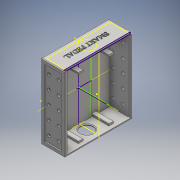
# Autodesk Inventor part: Part4
Saved by Autodesk Inventor 2016 (Build 200138000, 138)
## iProperties
Created: 2017-05-13
Part Number: Part4
Material: Generic
Document SubType Name: Modeling
Designer: ALIREZA
Density: 1 g/cm^3
Appearance: Default
Author: ALIREZA
Autodesk Inventor part; units mm, degrees
ref_plane "YZ Plane" through (0, 0, 0) normal (1, 0, 0) x (0, 1, 0)
ref_plane "XZ Plane" through (0, 0, 0) normal (0, 1, 0) x (-1, 0, 0)
ref_plane "XY Plane" through (0, 0, 0) normal (0, 0, 1) x (1, 0, 0)
sketch "Sketch1" plane through (0, 0, 0) normal (1, 0, 0) x (0, 1, 0)
  line L0 (50, 55) -> (-50, 55)
  line L1 (-50, 55) -> (-50, -55)
  line L2 (-50, -55) -> (50, -55)
  line L3 (50, -55) -> (50, 55)
  line L4 (50, 55) -> (-50, -55) construction
  line L5 (-50, 55) -> (50, -55) construction
  point P0 (0, 0)
  dimension "d0" = 100
  dimension "d1" = 110
  constraints: 12 end point, 2 midpoint, 2 parallel, 1 horizontal, 1 perpendicular
  measures "d0" distance of L2.end L1.end
  measures "d1" distance of L1.end L0.end
extrude "Extrusion1" add sketch "Sketch1" along normal blind 35
fillet "Fillet1" radius 1 12 edges at (17.5, 50, 55) (35, 50, 0) (35, 0, 55) (0, 0, 55) (0, 50, 0) (17.5, 50, -55) (35, 0, -55) (35, -50, 0) (17.5, -50, 55) (0, -50, 0) (0, 0, -55) (17.5, -50, -55)
sketch "Sketch2" plane through (35, 0, 0) normal (1, 0, 0) x (0, 0, -1)
  line L0 (52.5, -46.5) -> (-52.5, -46.5)
  line L1 (-52.5, -46.5) -> (-52.5, 46.5)
  line L2 (-52.5, 46.5) -> (52.5, 46.5)
  line L3 (52.5, 46.5) -> (52.5, -46.5)
  line L4 (52.5, -46.5) -> (-52.5, 46.5) construction
  line L5 (-52.5, -46.5) -> (52.5, 46.5) construction
  point P0 (0, 0)
  dimension "d5" = 105
  dimension "d6" = 93
  constraints: 12 end point, 2 midpoint, 2 parallel, 1 horizontal, 1 perpendicular
  measures "d5" distance of L1.end L2.end
  measures "d6" distance of L0.end L1.end
extrude "Extrusion2" cut sketch "Sketch2" against normal blind 30
sketch "Sketch3" plane through (34, 49, -55) normal (0, 0, -1) x (-1, 0, 0)
  line L0 (33, -98) -> (0, -98) projected
  line L1 (0, 0) -> (33, 0) projected
  circle A0 centre (16.5, -49) radius 9.5
  line L2 (16.5, -49) -> (16.5, -11.5096)
  line L3 (16.5, -49) -> (16.5, -84.2474)
  point P0 (34, -49)
  dimension "d55" = 19
  constraints: 4 end point, 2 vertical, 1 centre point
  measures "d55" diameter of A0
extrude "Extrusion3" cut sketch "Sketch3" against normal blind 30
sketch "Sketch4" plane through (0, 0, 0) normal (-1, 0, 0) x (0, 0, 1)
  point P0 (0, 0)
sketch "Sketch5" plane through (0, 0, 0) normal (-1, 0, 0) x (0, 0, 1)
  line L0 (19.6047, -32.8429) -> (51.5381, -32.8429) construction
  line L1 (51.5381, -32.8429) -> (51.5381, -46.3843) construction
  line L2 (51.5381, -46.3843) -> (19.6047, -46.3843) construction
  line L3 (19.6047, -46.3843) -> (19.6047, -32.8429) construction
  line L4 (20.2753, -38.9429) -> (20.2753, -32.8429)
  line L5 (20.2753, -32.8429) -> (21.532, -32.8429)
  line L6 (21.532, -32.8429) -> (21.532, -38.9429)
  line L7 (21.532, -38.9429) -> (20.2753, -38.9429)
  line L8 (22.8434, -38.9429) -> (22.8434, -32.8429)
  line L9 (22.8434, -32.8429) -> (24.7013, -32.8429)
  line L10 (24.7013, -32.8429) -> (25.9183, -37.4874)
  line L11 (25.9183, -37.4874) -> (27.1154, -32.8429)
  line L12 (27.1154, -32.8429) -> (28.9782, -32.8429)
  line L13 (28.9782, -32.8429) -> (28.9782, -38.9429)
  line L14 (28.9782, -38.9429) -> (27.8009, -38.9429)
  line L15 (27.8009, -38.9429) -> (27.8009, -34.0251)
  line L16 (27.8009, -34.0251) -> (26.564, -38.9429)
  line L17 (26.564, -38.9429) -> (25.2775, -38.9429)
  line L18 (25.2775, -38.9429) -> (24.0207, -34.0251)
  line L19 (24.0207, -34.0251) -> (24.0207, -38.9429)
  line L20 (24.0207, -38.9429) -> (22.8434, -38.9429)
  line L21 (31.5066, -38.9429) -> (31.5066, -33.9307)
  line L22 (31.5066, -33.9307) -> (29.6985, -33.9307)
  line L23 (29.6985, -33.9307) -> (29.6985, -32.8429)
  line L24 (29.6985, -32.8429) -> (34.5616, -32.8429)
  line L25 (34.5616, -32.8429) -> (34.5616, -33.9307)
  line L26 (34.5616, -33.9307) -> (32.7634, -33.9307)
  line L27 (32.7634, -33.9307) -> (32.7634, -38.9429)
  line L28 (32.7634, -38.9429) -> (31.5066, -38.9429)
  line L29 (35.2868, -38.9429) -> (35.2868, -32.8429)
  line L30 (35.2868, -32.8429) -> (39.7178, -32.8429)
  line L31 (39.7178, -32.8429) -> (39.7178, -33.9059)
  line L32 (39.7178, -33.9059) -> (36.5237, -33.9059)
  line L33 (36.5237, -33.9059) -> (36.5237, -35.2074)
  line L34 (36.5237, -35.2074) -> (39.4446, -35.2074)
  line L35 (39.4446, -35.2074) -> (39.4446, -36.2505)
  line L36 (39.4446, -36.2505) -> (36.5237, -36.2505)
  line L37 (36.5237, -36.2505) -> (36.5237, -37.8153)
  line L38 (36.5237, -37.8153) -> (39.8668, -37.8153)
  line L39 (39.8668, -37.8153) -> (39.8668, -38.9429)
  line L40 (39.8668, -38.9429) -> (35.2868, -38.9429)
  line L41 (40.8255, -38.9429) -> (40.8255, -32.8429)
  line L42 (40.8255, -32.8429) -> (42.0823, -32.8429)
  line L43 (42.0823, -32.8429) -> (42.0823, -35.3465)
  line L44 (42.0823, -35.3465) -> (44.4666, -32.8429)
  line L45 (44.4666, -32.8429) -> (46.0364, -32.8429)
  line L46 (46.0364, -32.8429) -> (43.5973, -35.3117)
  line L47 (43.5973, -35.3117) -> (46.2549, -38.9429)
  line L48 (46.2549, -38.9429) -> (44.72, -38.9429)
  line L49 (44.72, -38.9429) -> (42.733, -36.1512)
  line L50 (42.733, -36.1512) -> (42.0823, -36.797)
  line L51 (42.0823, -36.797) -> (42.0823, -38.9429)
  line L52 (42.0823, -38.9429) -> (40.8255, -38.9429)
  point P0 (0, 0)
  constraints: 2 other
sketch "Sketch6" plane through (0, 0, 0) normal (-1, 0, 0) x (0, 0, 1)
  point P0 (0, 0)
sketch "Sketch7" plane through (0, 0, 0) normal (-1, 0, 0) x (0, 0, 1)
  point P0 (0, 0)
sketch "Sketch8" plane through (0, 0, 0) normal (-1, 0, 0) x (0, 0, 1)
  point P0 (0, 0)
emboss "Emboss1" sketch "Sketch5" operation add depth 0.5 direction (1, 0, 0)
sketch "Sketch9" plane through (1, -49, 55) normal (0, 0, 1) x (1, 0, 0)
  line L0 (19.7914, 80.3195) -> (19.7914, -11.2085) construction
  line L1 (19.7914, -11.2085) -> (-27.1496, -11.2085) construction
  line L2 (-27.1496, -11.2085) -> (-27.1496, 80.3195) construction
  line L3 (-27.1496, 80.3195) -> (19.7914, 80.3195) construction
  line L4 (19.7914, 76.1011) -> (17.6889, 76.1011)
  line L5 (17.6889, 76.1011) -> (17.6889, 76.2685)
  spline S0 degree 2 poles (17.6889, 76.2685) (18.2915, 76.3488) (19.008, 76.764) (19.4365, 77.5407) (19.4365, 77.9492) knots 0 0 0 1 2 3 3 3
  spline S1 degree 2 poles (19.4365, 77.9492) (19.4365, 78.4179) (18.8607, 79.0272) (18.4991, 79.0272) knots 0 0 0 1 2 2 2
  spline S2 degree 2 poles (18.4991, 79.0272) (18.2178, 79.0272) (17.9902, 78.8397) knots 0 0 0 1 1 1
  spline S3 degree 2 poles (17.9902, 78.8397) (17.6487, 78.5585) (17.0862, 77.5072) knots 0 0 0 1 1 1
  spline S4 degree 2 poles (17.0862, 77.5072) (16.6309, 76.6568) (16.1421, 76.0341) (15.4725, 75.6993) (15.1109, 75.6993) knots 0 0 0 1 2 3 3 3
  spline S5 degree 2 poles (15.1109, 75.6993) (14.4213, 75.6993) (13.4169, 76.7707) (13.4169, 77.6144) knots 0 0 0 1 2 2 2
  spline S6 degree 2 poles (13.4169, 77.6144) (13.4169, 77.8822) (13.457, 78.1099) knots 0 0 0 1 1 1
  spline S7 degree 2 poles (13.457, 78.1099) (13.4838, 78.2505) (13.7651, 79.1276) (13.7651, 79.2482) knots 0 0 0 1 2 2 2
  spline S8 degree 2 poles (13.7651, 79.2482) (13.7651, 79.3553) (13.6244, 79.4892) (13.4169, 79.516) knots 0 0 0 1 2 2 2
  line L6 (13.4169, 79.516) -> (13.4169, 79.6834)
  line L7 (13.4169, 79.6834) -> (15.506, 79.6834)
  line L8 (15.506, 79.6834) -> (15.506, 79.516)
  spline S9 degree 2 poles (15.506, 79.516) (14.8498, 79.4022) (14.2003, 79.0071) (13.7651, 78.1969) (13.7651, 77.7081) knots 0 0 0 1 2 3 3 3
  spline S10 degree 2 poles (13.7651, 77.7081) (13.7651, 77.1523) (14.3677, 76.4961) (14.7627, 76.4961) knots 0 0 0 1 2 2 2
  spline S11 degree 2 poles (14.7627, 76.4961) (14.9904, 76.4961) (15.4524, 76.7439) (15.6466, 77.005) knots 0 0 0 1 2 2 2
  spline S12 degree 2 poles (15.6466, 77.005) (15.7805, 77.1791) (16.6577, 78.7393) (17.18, 79.4022) (17.8094, 79.7437) (18.1844, 79.7437) knots 0 0 0 1 2 3 4 4 4
  spline S13 degree 2 poles (18.1844, 79.7437) (18.8406, 79.7437) (19.7914, 78.7393) (19.7914, 77.9626) knots 0 0 0 1 2 2 2
  spline S14 degree 2 poles (19.7914, 77.9626) (19.7914, 77.4737) (19.557, 76.9314) knots 0 0 0 1 1 1
  spline S15 degree 2 poles (19.557, 76.9314) (19.4365, 76.6769) (19.4365, 76.5765) knots 0 0 0 1 1 1
  spline S16 degree 2 poles (19.4365, 76.5765) (19.4365, 76.456) (19.5771, 76.3154) (19.7914, 76.2685) knots 0 0 0 1 2 2 2
  line L9 (19.7914, 76.2685) -> (19.7914, 76.1011)
  line L10 (13.5575, 71.4273) -> (18.6866, 73.7843)
  line L11 (18.6866, 73.7843) -> (14.6154, 73.7843)
  spline S17 degree 2 poles (14.6154, 73.7843) (14.053, 73.7843) (13.9124, 73.6638) knots 0 0 0 1 1 1
  spline S18 degree 2 poles (13.9124, 73.6638) (13.7249, 73.4964) (13.7249, 73.1415) knots 0 0 0 1 1 1
  line L12 (13.7249, 73.1415) -> (13.7249, 72.9205)
  line L13 (13.7249, 72.9205) -> (13.5575, 72.9205)
  line L14 (13.5575, 72.9205) -> (13.5575, 75.0431)
  line L15 (13.5575, 75.0431) -> (13.7249, 75.0431)
  line L16 (13.7249, 75.0431) -> (13.7249, 74.8289)
  spline S19 degree 2 poles (13.7249, 74.8289) (13.7249, 74.4405) (13.9592, 74.2798) knots 0 0 0 1 1 1
  spline S20 degree 2 poles (13.9592, 74.2798) (14.1065, 74.1793) (14.6154, 74.1793) knots 0 0 0 1 1 1
  line L17 (14.6154, 74.1793) -> (18.5995, 74.1793)
  spline S21 degree 2 poles (18.5995, 74.1793) (19.0013, 74.1793) (19.1754, 74.2731) knots 0 0 0 1 1 1
  spline S22 degree 2 poles (19.1754, 74.2731) (19.3093, 74.3334) (19.4834, 74.6682) (19.4834, 75.0431) knots 0 0 0 1 2 2 2
  line L18 (19.4834, 75.0431) -> (19.6575, 75.0431)
  line L19 (19.6575, 75.0431) -> (19.6575, 73.3156)
  line L20 (19.6575, 73.3156) -> (14.8833, 71.1059)
  line L21 (14.8833, 71.1059) -> (19.6575, 68.9297)
  line L22 (19.6575, 68.9297) -> (19.6575, 67.2089)
  line L23 (19.6575, 67.2089) -> (19.4834, 67.2089)
  line L24 (19.4834, 67.2089) -> (19.4834, 67.4164)
  spline S23 degree 2 poles (19.4834, 67.4164) (19.4834, 67.8115) (19.2557, 67.9655) knots 0 0 0 1 1 1
  spline S24 degree 2 poles (19.2557, 67.9655) (19.1084, 68.066) (18.5995, 68.066) knots 0 0 0 1 1 1
  line L25 (18.5995, 68.066) -> (14.6154, 68.066)
  spline S25 degree 2 poles (14.6154, 68.066) (14.053, 68.066) (13.9124, 67.9454) knots 0 0 0 1 1 1
  spline S26 degree 2 poles (13.9124, 67.9454) (13.7249, 67.778) (13.7249, 67.4164) knots 0 0 0 1 1 1
  line L26 (13.7249, 67.4164) -> (13.7249, 67.2089)
  line L27 (13.7249, 67.2089) -> (13.5575, 67.2089)
  line L28 (13.5575, 67.2089) -> (13.5575, 69.8002)
  line L29 (13.5575, 69.8002) -> (13.7249, 69.8002)
  line L30 (13.7249, 69.8002) -> (13.7249, 69.5792)
  spline S27 degree 2 poles (13.7249, 69.5792) (13.7249, 69.1842) (13.9592, 69.0302) knots 0 0 0 1 1 1
  spline S28 degree 2 poles (13.9592, 69.0302) (14.1065, 68.9297) (14.6154, 68.9297) knots 0 0 0 1 1 1
  line L31 (14.6154, 68.9297) -> (18.6866, 68.9297)
  line L32 (18.6866, 68.9297) -> (13.5575, 71.2867)
  line L33 (13.5575, 71.2867) -> (13.5575, 71.4273)
  line L34 (15.593, 62.8029) -> (15.593, 65.1599)
  line L35 (15.593, 65.1599) -> (14.6355, 65.5751)
  spline S29 degree 2 poles (14.6355, 65.5751) (14.2806, 65.7291) (14.1065, 65.7291) knots 0 0 0 1 1 1
  spline S30 degree 2 poles (14.1065, 65.7291) (13.9659, 65.7291) (13.7517, 65.4612) (13.7249, 65.026) knots 0 0 0 1 2 2 2
  line L36 (13.7249, 65.026) -> (13.5575, 65.026)
  line L37 (13.5575, 65.026) -> (13.5575, 66.9477)
  line L38 (13.5575, 66.9477) -> (13.7249, 66.9477)
  spline S31 degree 2 poles (13.7249, 66.9477) (13.7918, 66.5594) (13.899, 66.4455) knots 0 0 0 1 1 1
  spline S32 degree 2 poles (13.899, 66.4455) (14.1132, 66.2179) (14.7761, 65.9433) knots 0 0 0 1 1 1
  line L39 (14.7761, 65.9433) -> (19.7914, 63.8006)
  line L40 (19.7914, 63.8006) -> (19.7914, 63.6399)
  line L41 (19.7914, 63.6399) -> (14.7159, 61.5173)
  spline S33 degree 2 poles (14.7159, 61.5173) (14.1065, 61.2629) (13.7517, 60.841) (13.7249, 60.4728) knots 0 0 0 1 2 2 2
  line L42 (13.7249, 60.4728) -> (13.5575, 60.4728)
  line L43 (13.5575, 60.4728) -> (13.5575, 62.8766)
  line L44 (13.5575, 62.8766) -> (13.7249, 62.8766)
  spline S34 degree 2 poles (13.7249, 62.8766) (13.745, 62.5083) (13.9458, 62.2539) (14.0998, 62.2539) knots 0 0 0 1 2 2 2
  spline S35 degree 2 poles (14.0998, 62.2539) (14.294, 62.2539) (14.7159, 62.4347) knots 0 0 0 1 1 1
  line L45 (14.7159, 62.4347) -> (15.593, 62.8029)
  line L46 (15.9345, 62.9235) -> (18.3919, 63.9613)
  line L47 (18.3919, 63.9613) -> (15.9345, 65.026)
  line L48 (15.9345, 65.026) -> (15.9345, 62.9235)
  line L49 (13.5575, 54.1451) -> (13.5575, 55.7722)
  line L50 (13.5575, 55.7722) -> (16.4099, 57.8346)
  spline S36 degree 2 poles (16.4099, 57.8346) (16.3966, 58.0689) (16.3966, 58.2028) knots 0 0 0 1 1 1
  spline S37 degree 2 poles (16.3966, 58.2028) (16.3966, 58.2698) (16.4032, 58.4037) (16.4099, 58.4707) knots 0 0 0 1 2 2 2
  line L51 (16.4099, 58.4707) -> (14.6355, 58.4707)
  spline S38 degree 2 poles (14.6355, 58.4707) (14.0597, 58.4707) (13.9258, 58.3435) knots 0 0 0 1 1 1
  spline S39 degree 2 poles (13.9258, 58.3435) (13.7249, 58.1761) (13.7249, 57.8346) knots 0 0 0 1 1 1
  line L52 (13.7249, 57.8346) -> (13.7249, 57.5935)
  line L53 (13.7249, 57.5935) -> (13.5575, 57.5935)
  line L54 (13.5575, 57.5935) -> (13.5575, 60.2116)
  line L55 (13.5575, 60.2116) -> (13.7249, 60.2116)
  line L56 (13.7249, 60.2116) -> (13.7249, 59.9773)
  spline S40 degree 2 poles (13.7249, 59.9773) (13.7249, 59.5956) (13.9726, 59.4282) knots 0 0 0 1 1 1
  spline S41 degree 2 poles (13.9726, 59.4282) (14.1132, 59.3345) (14.6355, 59.3345) knots 0 0 0 1 1 1
  line L57 (14.6355, 59.3345) -> (18.5727, 59.3345)
  spline S42 degree 2 poles (18.5727, 59.3345) (19.1486, 59.3345) (19.2892, 59.4617) knots 0 0 0 1 1 1
  spline S43 degree 2 poles (19.2892, 59.4617) (19.4834, 59.6358) (19.4834, 59.9773) knots 0 0 0 1 1 1
  line L58 (19.4834, 59.9773) -> (19.4834, 60.2116)
  line L59 (19.4834, 60.2116) -> (19.6575, 60.2116)
  line L60 (19.6575, 60.2116) -> (19.6575, 57.9886)
  spline S44 degree 2 poles (19.6575, 57.9886) (19.6575, 57.0177) (19.3696, 56.1003) (18.6062, 55.4508) (18.0839, 55.4508) knots 0 0 0 1 2 3 3 3
  spline S45 degree 2 poles (18.0839, 55.4508) (17.5215, 55.4508) (16.6912, 56.1874) (16.5238, 56.9574) knots 0 0 0 1 2 2 2
  line L61 (16.5238, 56.9574) -> (14.7761, 55.6986)
  spline S46 degree 2 poles (14.7761, 55.6986) (14.1735, 55.27) (13.7784, 54.6473) (13.7249, 54.1451) knots 0 0 0 1 2 2 2
  line L62 (13.7249, 54.1451) -> (13.5575, 54.1451)
  spline S47 degree 2 poles (16.6845, 58.4707) (16.6845, 58.3836) (16.6845, 58.2631) (16.6845, 58.2229) knots 0 0 0 1 2 2 2
  spline S48 degree 2 poles (16.6845, 58.2229) (16.6845, 57.3525) (17.4411, 56.4619) (18.0237, 56.4619) knots 0 0 0 1 2 2 2
  spline S49 degree 2 poles (18.0237, 56.4619) (18.5995, 56.4619) (19.3093, 57.1784) (19.3093, 57.7676) knots 0 0 0 1 2 2 2
  spline S50 degree 2 poles (19.3093, 57.7676) (19.3093, 58.0287) (19.2222, 58.4707) knots 0 0 0 1 1 1
  line L63 (19.2222, 58.4707) -> (16.6845, 58.4707)
  line L64 (19.6575, 48.9022) -> (18.2178, 48.8285)
  line L65 (18.2178, 48.8285) -> (18.2178, 49.0026)
  spline S51 degree 2 poles (18.2178, 49.0026) (18.5995, 49.0495) (18.7602, 49.1365) knots 0 0 0 1 1 1
  spline S52 degree 2 poles (18.7602, 49.1365) (19.0214, 49.2772) (19.2691, 49.7459) (19.2691, 50.1208) knots 0 0 0 1 2 2 2
  line L66 (19.2691, 50.1208) -> (19.2691, 50.9712)
  line L67 (19.2691, 50.9712) -> (14.6154, 50.9712)
  spline S53 degree 2 poles (14.6154, 50.9712) (14.053, 50.9712) (13.9124, 50.8507) knots 0 0 0 1 1 1
  spline S54 degree 2 poles (13.9124, 50.8507) (13.7249, 50.6833) (13.7249, 50.3284) knots 0 0 0 1 1 1
  line L68 (13.7249, 50.3284) -> (13.7249, 50.1208)
  line L69 (13.7249, 50.1208) -> (13.5575, 50.1208)
  line L70 (13.5575, 50.1208) -> (13.5575, 52.7055)
  line L71 (13.5575, 52.7055) -> (13.7249, 52.7055)
  line L72 (13.7249, 52.7055) -> (13.7249, 52.4845)
  spline S55 degree 2 poles (13.7249, 52.4845) (13.7249, 52.1028) (13.9592, 51.9354) knots 0 0 0 1 1 1
  spline S56 degree 2 poles (13.9592, 51.9354) (14.1065, 51.8417) (14.6154, 51.8417) knots 0 0 0 1 1 1
  line L73 (14.6154, 51.8417) -> (19.2691, 51.8417)
  line L74 (19.2691, 51.8417) -> (19.2691, 52.5716)
  spline S57 degree 2 poles (19.2691, 52.5716) (19.2691, 53.0001) (19.2088, 53.1809) knots 0 0 0 1 1 1
  spline S58 degree 2 poles (19.2088, 53.1809) (19.1218, 53.4152) (18.6397, 53.7433) (18.2178, 53.7768) knots 0 0 0 1 2 2 2
  line L75 (18.2178, 53.7768) -> (18.2178, 53.9442)
  line L76 (18.2178, 53.9442) -> (19.6575, 53.8773)
  line L77 (19.6575, 53.8773) -> (19.6575, 48.9022)
  line L78 (16.4099, 44.4226) -> (14.6355, 44.4226)
  spline S59 degree 2 poles (14.6355, 44.4226) (14.0597, 44.4226) (13.9258, 44.2954) knots 0 0 0 1 1 1
  spline S60 degree 2 poles (13.9258, 44.2954) (13.7249, 44.128) (13.7249, 43.7798) knots 0 0 0 1 1 1
  line L79 (13.7249, 43.7798) -> (13.7249, 43.5454)
  line L80 (13.7249, 43.5454) -> (13.5575, 43.5454)
  line L81 (13.5575, 43.5454) -> (13.5575, 46.1568)
  line L82 (13.5575, 46.1568) -> (13.7249, 46.1568)
  line L83 (13.7249, 46.1568) -> (13.7249, 45.9292)
  spline S61 degree 2 poles (13.7249, 45.9292) (13.7249, 45.5475) (13.9726, 45.3734) knots 0 0 0 1 1 1
  spline S62 degree 2 poles (13.9726, 45.3734) (14.1132, 45.2864) (14.6355, 45.2864) knots 0 0 0 1 1 1
  line L84 (14.6355, 45.2864) -> (18.5727, 45.2864)
  spline S63 degree 2 poles (18.5727, 45.2864) (19.1486, 45.2864) (19.2892, 45.4069) knots 0 0 0 1 1 1
  spline S64 degree 2 poles (19.2892, 45.4069) (19.4834, 45.5877) (19.4834, 45.9292) knots 0 0 0 1 1 1
  line L85 (19.4834, 45.9292) -> (19.4834, 46.1568)
  line L86 (19.4834, 46.1568) -> (19.6575, 46.1568)
  line L87 (19.6575, 46.1568) -> (19.6575, 43.9271)
  spline S65 degree 2 poles (19.6575, 43.9271) (19.6575, 43.1035) (19.3093, 42.1661) (18.5192, 41.5166) (17.9634, 41.5166) knots 0 0 0 1 2 3 3 3
  spline S66 degree 2 poles (17.9634, 41.5166) (17.2202, 41.5166) (16.2894, 42.5009) (16.2894, 43.3981) knots 0 0 0 1 2 2 2
  spline S67 degree 2 poles (16.2894, 43.3981) (16.2894, 43.6191) (16.3497, 44.1347) (16.4099, 44.4226) knots 0 0 0 1 2 2 2
  spline S68 degree 2 poles (16.6711, 44.4226) (16.6242, 44.1882) (16.5773, 43.8133) (16.5773, 43.686) knots 0 0 0 1 2 2 2
  spline S69 degree 2 poles (16.5773, 43.686) (16.5773, 43.2173) (17.3005, 42.541) (17.8764, 42.541) knots 0 0 0 1 2 2 2
  spline S70 degree 2 poles (17.8764, 42.541) (18.2714, 42.541) (18.9544, 42.8624) (19.2892, 43.4584) (19.2892, 43.84) knots 0 0 0 1 2 3 3 3
  spline S71 degree 2 poles (19.2892, 43.84) (19.2892, 44.061) (19.2022, 44.4226) knots 0 0 0 1 1 1
  line L88 (19.2022, 44.4226) -> (16.6711, 44.4226)
  line L89 (19.316, 39.2667) -> (16.9054, 39.2667)
  line L90 (16.9054, 39.2667) -> (16.9054, 37.9275)
  spline S72 degree 2 poles (16.9054, 37.9275) (16.9054, 37.4053) (17.0661, 37.2312) knots 0 0 0 1 1 1
  spline S73 degree 2 poles (17.0661, 37.2312) (17.2737, 36.9968) (17.796, 36.97) knots 0 0 0 1 1 1
  line L91 (17.796, 36.97) -> (17.796, 36.8026)
  line L92 (17.796, 36.8026) -> (15.6801, 36.8026)
  line L93 (15.6801, 36.8026) -> (15.6801, 36.97)
  spline S74 degree 2 poles (15.6801, 36.97) (16.1153, 37.0303) (16.2492, 37.0972) knots 0 0 0 1 1 1
  spline S75 degree 2 poles (16.2492, 37.0972) (16.4032, 37.1776) (16.584, 37.5392) (16.584, 37.9275) knots 0 0 0 1 2 2 2
  line L94 (16.584, 37.9275) -> (16.584, 39.2667)
  line L95 (16.584, 39.2667) -> (14.5753, 39.2667)
  spline S76 degree 2 poles (14.5753, 39.2667) (14.1668, 39.2667) (13.9927, 39.1931) (13.8856, 39.0123) (13.8856, 38.7645) knots 0 0 0 1 2 3 3 3
  line L96 (13.8856, 38.7645) -> (13.8856, 37.7267)
  spline S77 degree 2 poles (13.8856, 37.7267) (13.8856, 37.2111) (14.0329, 36.7491) (14.2405, 36.5281) knots 0 0 0 1 2 2 2
  spline S78 degree 2 poles (14.2405, 36.5281) (14.5217, 36.2469) (15.0841, 35.9589) knots 0 0 0 1 1 1
  line L97 (15.0841, 35.9589) -> (15.0841, 35.7781)
  line L98 (15.0841, 35.7781) -> (13.5575, 36.3071)
  line L99 (13.5575, 36.3071) -> (13.5575, 40.9943)
  line L100 (13.5575, 40.9943) -> (13.7249, 40.9943)
  line L101 (13.7249, 40.9943) -> (13.7249, 40.78)
  spline S79 degree 2 poles (13.7249, 40.78) (13.7249, 40.5657) (13.8253, 40.3782) knots 0 0 0 1 1 1
  spline S80 degree 2 poles (13.8253, 40.3782) (13.899, 40.2309) (14.1869, 40.1238) (14.6288, 40.1238) knots 0 0 0 1 2 2 2
  line L102 (14.6288, 40.1238) -> (18.5928, 40.1238)
  spline S81 degree 2 poles (18.5928, 40.1238) (19.1754, 40.1238) (19.3093, 40.2443) knots 0 0 0 1 1 1
  spline S82 degree 2 poles (19.3093, 40.2443) (19.4834, 40.405) (19.4834, 40.78) knots 0 0 0 1 1 1
  line L103 (19.4834, 40.78) -> (19.4834, 40.9943)
  line L104 (19.4834, 40.9943) -> (19.6575, 40.9943)
  line L105 (19.6575, 40.9943) -> (19.6575, 36.3071)
  line L106 (19.6575, 36.3071) -> (18.3183, 36.2335)
  line L107 (18.3183, 36.2335) -> (18.3183, 36.4076)
  spline S83 degree 2 poles (18.3183, 36.4076) (18.7937, 36.5013) (19.1553, 36.7357) (19.2557, 36.9633) knots 0 0 0 1 2 2 2
  spline S84 degree 2 poles (19.2557, 36.9633) (19.316, 37.1441) (19.316, 37.5927) knots 0 0 0 1 1 1
  line L108 (19.316, 37.5927) -> (19.316, 39.2667)
  line L109 (13.5575, 35.4166) -> (13.7249, 35.4166)
  line L110 (13.7249, 35.4166) -> (13.7249, 35.1822)
  spline S85 degree 2 poles (13.7249, 35.1822) (13.7249, 34.8005) (13.9726, 34.6331) knots 0 0 0 1 1 1
  spline S86 degree 2 poles (13.9726, 34.6331) (14.1199, 34.5394) (14.6355, 34.5394) knots 0 0 0 1 1 1
  line L111 (14.6355, 34.5394) -> (18.5727, 34.5394)
  spline S87 degree 2 poles (18.5727, 34.5394) (19.1419, 34.5394) (19.2892, 34.6666) knots 0 0 0 1 1 1
  spline S88 degree 2 poles (19.2892, 34.6666) (19.4834, 34.8407) (19.4834, 35.1822) knots 0 0 0 1 1 1
  line L112 (19.4834, 35.1822) -> (19.4834, 35.4166)
  line L113 (19.4834, 35.4166) -> (19.6575, 35.4166)
  line L114 (19.6575, 35.4166) -> (19.6575, 32.9324)
  spline S89 degree 2 poles (19.6575, 32.9324) (19.6575, 31.5664) (19.0348, 30.1402) (17.5884, 29.2764) (16.6376, 29.2764) knots 0 0 0 1 2 3 3 3
  spline S90 degree 2 poles (16.6376, 29.2764) (15.3654, 29.2764) (14.5083, 30.0464) knots 0 0 0 1 1 1
  spline S91 degree 2 poles (14.5083, 30.0464) (13.5575, 30.9169) (13.5575, 32.6913) knots 0 0 0 1 1 1
  line L115 (13.5575, 32.6913) -> (13.5575, 35.4166)
  spline S92 degree 2 poles (13.9994, 33.6689) (13.8722, 33.0998) (13.8722, 32.7181) knots 0 0 0 1 1 1
  spline S93 degree 2 poles (13.8722, 32.7181) (13.8722, 31.6735) (15.3386, 30.3009) (16.5907, 30.3009) knots 0 0 0 1 2 2 2
  spline S94 degree 2 poles (16.5907, 30.3009) (17.8563, 30.3009) (19.3093, 31.6735) (19.3093, 32.7516) knots 0 0 0 1 2 2 2
  spline S95 degree 2 poles (19.3093, 32.7516) (19.3093, 33.1533) (19.1754, 33.6689) knots 0 0 0 1 1 1
  line L116 (19.1754, 33.6689) -> (13.9994, 33.6689)
  line L117 (15.593, 24.7098) -> (15.593, 27.0667)
  line L118 (15.593, 27.0667) -> (14.6355, 27.4819)
  spline S96 degree 2 poles (14.6355, 27.4819) (14.2806, 27.6359) (14.1065, 27.6359) knots 0 0 0 1 1 1
  spline S97 degree 2 poles (14.1065, 27.6359) (13.9659, 27.6359) (13.7517, 27.368) (13.7249, 26.9328) knots 0 0 0 1 2 2 2
  line L119 (13.7249, 26.9328) -> (13.5575, 26.9328)
  line L120 (13.5575, 26.9328) -> (13.5575, 28.8545)
  line L121 (13.5575, 28.8545) -> (13.7249, 28.8545)
  spline S98 degree 2 poles (13.7249, 28.8545) (13.7918, 28.4662) (13.899, 28.3523) knots 0 0 0 1 1 1
  spline S99 degree 2 poles (13.899, 28.3523) (14.1132, 28.1247) (14.7761, 27.8501) knots 0 0 0 1 1 1
  line L122 (14.7761, 27.8501) -> (19.7914, 25.7074)
  line L123 (19.7914, 25.7074) -> (19.7914, 25.5467)
  line L124 (19.7914, 25.5467) -> (14.7159, 23.4241)
  spline S100 degree 2 poles (14.7159, 23.4241) (14.1065, 23.1697) (13.7517, 22.7478) (13.7249, 22.3796) knots 0 0 0 1 2 2 2
  line L125 (13.7249, 22.3796) -> (13.5575, 22.3796)
  line L126 (13.5575, 22.3796) -> (13.5575, 24.7834)
  line L127 (13.5575, 24.7834) -> (13.7249, 24.7834)
  spline S101 degree 2 poles (13.7249, 24.7834) (13.745, 24.4151) (13.9458, 24.1607) (14.0998, 24.1607) knots 0 0 0 1 2 2 2
  spline S102 degree 2 poles (14.0998, 24.1607) (14.294, 24.1607) (14.7159, 24.3415) knots 0 0 0 1 1 1
  line L128 (14.7159, 24.3415) -> (15.593, 24.7098)
  line L129 (15.9345, 24.8303) -> (18.3919, 25.8681)
  line L130 (18.3919, 25.8681) -> (15.9345, 26.9328)
  line L131 (15.9345, 26.9328) -> (15.9345, 24.8303)
  line L132 (15.2382, 16.996) -> (15.2114, 16.8487)
  line L133 (15.2114, 16.8487) -> (13.5575, 17.371)
  line L134 (13.5575, 17.371) -> (13.5575, 22.0849)
  line L135 (13.5575, 22.0849) -> (13.7249, 22.0849)
  line L136 (13.7249, 22.0849) -> (13.7249, 21.8573)
  spline S103 degree 2 poles (13.7249, 21.8573) (13.7249, 21.4689) (13.9726, 21.3082) knots 0 0 0 1 1 1
  spline S104 degree 2 poles (13.9726, 21.3082) (14.1199, 21.2078) (14.6422, 21.2078) knots 0 0 0 1 1 1
  line L137 (14.6422, 21.2078) -> (18.5727, 21.2078)
  spline S105 degree 2 poles (18.5727, 21.2078) (19.1419, 21.2078) (19.2892, 21.335) knots 0 0 0 1 1 1
  spline S106 degree 2 poles (19.2892, 21.335) (19.4834, 21.5091) (19.4834, 21.8573) knots 0 0 0 1 1 1
  line L138 (19.4834, 21.8573) -> (19.4834, 22.0849)
  line L139 (19.4834, 22.0849) -> (19.6575, 22.0849)
  line L140 (19.6575, 22.0849) -> (19.6575, 19.3262)
  line L141 (19.6575, 19.3262) -> (19.4834, 19.3262)
  spline S107 degree 2 poles (19.4834, 19.3262) (19.4901, 19.815) (19.3026, 20.2034) (19.0147, 20.3507) (18.4723, 20.3507) knots 0 0 0 1 2 3 3 3
  line L142 (18.4723, 20.3507) -> (14.6422, 20.3507)
  spline S108 degree 2 poles (14.6422, 20.3507) (14.2672, 20.3507) (14.1266, 20.277) knots 0 0 0 1 1 1
  spline S109 degree 2 poles (14.1266, 20.277) (14.0329, 20.2235) (13.9458, 19.9958) (13.9458, 19.4066) knots 0 0 0 1 2 2 2
  line L143 (13.9458, 19.4066) -> (13.9458, 18.9646)
  spline S110 degree 2 poles (13.9458, 18.9646) (13.9458, 18.2683) (14.1467, 17.6991) (14.6757, 17.2304) (15.2382, 16.996) knots 0 0 0 1 2 3 3 3
  point P0 (-1, 49)
  constraints: 2 other
emboss "Emboss2" sketch "Sketch9" operation add depth 0.5 direction (0, 0, -1)
sketch "Sketch10" plane through (1, -50, -54) normal (0, -1, 0) x (1, 0, 0)
  circle A0 centre (23.8045, 92.5062) radius 2.2175
  line L0 (23.8045, 92.5062) -> (31.7537, 92.5062)
  line L1 (31.7537, 92.5062) -> (18.4963, 92.5062)
  line L2 (18.4963, 92.5062) -> (23.8045, 92.5062)
  line L3 (24.7351, 104.1704) -> (24.7351, 90.393)
  line L4 (0, 108) -> (33, 108) projected
  circle A1 centre (23.8045, 72.9922) radius 2.2175
  circle A2 centre (23.8045, 53.4782) radius 2.2175
  circle A3 centre (23.8045, 33.9642) radius 2.2175
  circle A4 centre (23.8045, 14.4502) radius 2.2175
  circle A5 centre (9.1955, 92.5062) radius 2.2175
  circle A6 centre (9.1955, 72.9922) radius 2.2175
  circle A7 centre (9.1955, 53.4782) radius 2.2175
  circle A8 centre (9.1955, 33.9642) radius 2.2175
  circle A9 centre (9.1955, 14.4502) radius 2.2175
  line L5 (0, 0) -> (0, 108) projected
  line L6 (33, 108) -> (33, 0) projected
  line L7 (29, 103.2061) -> (4, 4.7939) construction
  line L8 (5.4125, 97.6458) -> (27.5875, 10.3542) construction
  point P0 (-1, 54)
  point P1 (16.5, 54)
  dimension "d15" = 4.435
  dimension "d26" = 19.514
  dimension "d33" = 19.514
  constraints: 12 end point, 10 centre point, 2 midpoint, 1 collinear, 1 horizontal, 1 perpendicular, 1 point on line, 1 vertical, 8 other
  measures "d15" diameter of A0
  measures "d26" distance of L0.start A1.centre
  measures "d33" distance of A6.centre A5.centre
extrude "Extrusion4" cut sketch "Sketch10" against normal blind 200
sketch "Sketch11" plane through (1, -50, -54) normal (0, -1, 0) x (1, 0, 0)
  point P0 (-1, 54)
sketch "Sketch12" plane through (1, -50, -54) normal (0, -1, 0) x (1, 0, 0)
  point P0 (-1, 54)
sketch "Sketch13" plane through (1, -50, -54) normal (0, -1, 0) x (1, 0, 0)
  point P0 (-1, 54)
sketch "Sketch14" plane through (35, -46.5, 52.5) normal (0, 1, 0) x (1, 0, 0)
  point P0 (-35, 52.5)
sketch "Sketch15" plane through (1, 50, 54) normal (0, 1, 0) x (1, 0, 0)
  line L0 (33, 108) -> (0, 108) projected
  line L1 (0, 108) -> (0, 0) projected
  line L2 (33, 108) -> (0, 108)
  line L3 (0, 108) -> (0, 0)
  line L4 (0, 0) -> (33, 0)
  line L5 (33, 0) -> (33, 108)
  line L6 (4, 106.5) -> (4, 1.5) projected
  line L7 (29, 103.6928) -> (4, 103.6928)
  line L8 (4, 103.6928) -> (4, 4.3072)
  line L9 (4, 4.3072) -> (29, 4.3072)
  line L10 (29, 4.3072) -> (29, 103.6928)
  line L11 (29, 103.6928) -> (4, 4.3072) construction
  line L12 (4, 103.6928) -> (29, 4.3072) construction
  point P0 (-1, 54)
  point P1 (16.5, 54)
  constraints: 20 end point, 4 parallel, 2 horizontal, 2 midpoint, 2 perpendicular, 1 point on line
extrude "Extrusion5" cut sketch "Sketch15" against normal blind 1.5 contours L7 L10 L9 L6
sketch "Sketch16" plane through (1, 48.5, 54) normal (0, 1, 0) x (1, 0, 0)
  point P0 (-1, 54)
sketch "Sketch17" plane through (5, 0, 0) normal (1, 0, 0) x (0, 0, -1)
  point P0 (0, 0)
sketch "Sketch18" plane through (5, 0, 0) normal (1, 0, 0) x (0, 0, -1)
  line L0 (52.5, -9.5) -> (52.5, 9.5) projected
  line L1 (52.5, 0) -> (-52.5, 0)
  line L2 (-52.5, -46.5) -> (-52.5, 46.5) projected
  point P0 (0, 0)
  constraints: 2 end point, 2 midpoint
ref_plane "Work Plane1" through (5, 0, -52.5) normal (0, 1, 0) x (0, 0, 1)
mirror "Mirror1" about plane through (5, 0, -52.5) normal (0, 1, 0) of "Extrusion5"
ref_plane "Work Plane2" through (2.5, 0, 0) normal (1, 0, 0) x (0, 0, -1)
ref_plane "Work Plane3" through (17.5, -49, 55) normal (1, 0, 0) x (0, 0, -1)
pattern_of_nothing "Mirror2"
sketch "Sketch19" plane through (1, -49, 55) normal (0, 0, 1) x (1, 0, 0)
  point P0 (-1, 49)
sketch "Sketch20" plane through (1, -49, 55) normal (0, 0, 1) x (1, 0, 0)
  point P0 (-1, 49)
sketch "Sketch21" plane through (32.5, 0, 0) normal (-1, 0, 0) x (0, 0, -1)
  point P0 (0, 0)
sketch "Sketch22" plane through (1, -49, 55) normal (0, 0, 1) x (1, 0, 0)
  point P0 (-1, 49)
sketch "Sketch23" plane through (1, -49, 55) normal (0, 0, 1) x (1, 0, 0)
  line L0 (33, 98) -> (0, 98) projected
  line L1 (0, 0) -> (33, 0) projected
  line L2 (33, 98) -> (31.1, 98)
  line L3 (31.1, 98) -> (31.1, 0)
  line L4 (31.1, 0) -> (33, 0)
  line L5 (33, 0) -> (33, 98)
  point P0 (-1, 49)
  dimension "d37" = 1.9
  constraints: 8 end point, 2 parallel, 1 horizontal, 1 perpendicular, 1 point on line
  measures "d37" distance of L4.end L3.end
extrude "Extrusion6" cut sketch "Sketch23" against normal up to surface (107.5 mm away)
sketch "Sketch24" plane through (35, 46.5, -52.5) normal (0, -1, 0) x (1, 0, 0)
  point P0 (-35, 52.5)
sketch "Sketch25" plane through (1, -49, 55) normal (0, 0, 1) x (1, 0, 0)
  point P0 (-1, 49)
sketch "Sketch26" plane through (1, -49, 55) normal (0, 0, 1) x (1, 0, 0)
  line L0 (34, 0) -> (34, 98) projected
  line L1 (31.1, 95.5) -> (31.1, 2.5) projected
  line L2 (34, 95.5519) -> (31.1, 95.5519)
  line L3 (31.1, 95.5519) -> (31.1, 2.5)
  line L4 (31.1, 2.5) -> (34, 2.5)
  line L5 (34, 2.5) -> (34, 95.5519)
  point P0 (-1, 49)
  constraints: 8 end point, 2 parallel, 1 horizontal, 1 perpendicular, 1 point on line
extrude "Extrusion7" cut sketch "Sketch26" against normal up to surface (107.5 mm away)
sketch "Sketch27" plane through (1, -49, 55) normal (0, 0, 1) x (1, 0, 0)
  line L0 (33, 98) -> (33, 95.5519) projected
  line L1 (33, 95.5519) -> (33, 98)
  line L2 (33, 98) -> (31.1, 98)
  line L3 (31.1, 0) -> (31.1, 98) projected
  line L4 (31.1, 98) -> (31.1, 0)
  line L5 (31.1, 0) -> (33, 0)
  line L6 (33, 2.5) -> (33, 0) projected
  line L7 (33, 0) -> (33, 2.5)
  line L8 (33, 2.5) -> (34, 2.5)
  line L9 (34, 95.5519) -> (34, 98) projected
  line L10 (34, 2.5) -> (34, 95.5519)
  line L11 (34, 95.5519) -> (33, 95.5519)
  point P0 (-1, 49)
  constraints: 16 end point, 7 perpendicular, 1 point on line, 1 vertical
sketch "Sketch28" plane through (1, -49, 55) normal (0, 0, 1) x (1, 0, 0)
  point P0 (-1, 49)
sketch "Sketch29" plane through (5, 46.5, -52.5) normal (0, -1, 0) x (1, 0, 0)
  point P0 (-5, 52.5)
sketch "Sketch30" plane through (32.1, -49, 55) normal (1, 0, 0) x (0, 0, -1)
  point P0 (55, 49)
sketch "Sketch31" plane through (5, 0, 0) normal (1, 0, 0) x (0, 0, -1)
  line L0 (52.5, -9.5) -> (52.5, 9.5) projected
  line L1 (52.5, 0) -> (-42.5, 0)
  line L2 (-42.5, 0) -> (-42.5, -22.5)
  line L3 (-42.5, 0) -> (-42.5, 22.5)
  line L4 (52.5, 0) -> (52.5, -22.5)
  line L5 (52.5, 46.5) -> (52.5, -46.5) projected
  line L6 (52.5, 0) -> (52.5, 22.5)
  line L7 (52.5, -21.7139) -> (51.5, -21.7139)
  line L8 (47.9452, -19.0051) -> (50.9452, -19.0051)
  line L9 (50.9452, -19.0051) -> (50.9452, -26.0051)
  line L10 (50.9452, -26.0051) -> (47.9452, -26.0051)
  line L11 (47.9452, -26.0051) -> (47.9452, -19.0051)
  line L12 (47.9452, -19.0051) -> (50.9452, -26.0051) construction
  line L13 (50.9452, -19.0051) -> (47.9452, -26.0051) construction
  point P0 (0, 0)
  point P1 (49.4452, -22.5051)
  dimension "d42" = 95
  dimension "d43" = 22.5
  dimension "d44" = 22.5
  dimension "d45" = 22.5
  dimension "d46" = 22.5
  dimension "d48" = 1
  dimension "d51" = 3
  dimension "d52" = 7
  constraints: 24 end point, 3 midpoint, 3 point on line, 2 horizontal, 2 parallel, 2 perpendicular, 2 vertical
  measures "d42" distance of L1.start L1.end
  measures "d43" distance of L1.end L2.end
  measures "d44" distance of L1.end L3.end
  measures "d45" distance of L1.start L4.end
  measures "d46" distance of L1.start L6.end
  measures "d48" distance of L7.start L7.end
  measures "d51" distance of L9.end L10.end
  measures "d52" distance of L8.end L9.end
extrude "Extrusion8" add sketch "Sketch31" along normal blind 26
sketch "Sketch32" plane through (5, -46.5, -52.5) normal (0, 0, 1) x (1, 0, 0)
  point P0 (-5, 46.5)
fillet "Fillet2" radius 1 2 edges at (27, 0, -52.5) (27, 0, -55)
sketch "Sketch33" plane through (5, -26.0051, -47.9452) normal (0, 0, 1) x (1, 0, 0)
  point P0 (-5, 26.0051)
sketch "Sketch34" plane through (5, 0, 0) normal (1, 0, 0) x (0, 0, -1)
  point P0 (0, 0)
sketch "Sketch35" plane through (31, -26.0051, -50.9452) normal (0, 0, -1) x (-1, 0, 0)
  line L0 (0, 7) -> (0, 0) projected
  line L1 (0, 3.5) -> (25.2568, 3.5)
  line L2 (13.4936, 0) -> (13.4936, 6.0578)
  line L3 (9.9936, 3) -> (16.9936, 3)
  line L4 (16.9936, 3) -> (16.9936, 4)
  line L5 (16.9936, 4) -> (9.9936, 4)
  line L6 (9.9936, 4) -> (9.9936, 3)
  line L7 (9.9936, 3) -> (16.9936, 4) construction
  line L8 (16.9936, 3) -> (9.9936, 4) construction
  point P0 (31, 26.0051)
  point P1 (13.4936, 3.5)
  dimension "d59" = 7
  dimension "d60" = 1
  constraints: 16 end point, 3 midpoint, 2 horizontal, 2 parallel, 2 perpendicular, 2 point on line
  measures "d59" distance of L5.end L4.end
  measures "d60" distance of L4.end L3.end
extrude "Extrusion9" add sketch "Sketch35" along normal blind 0.7
fillet "Fillet5" radius 0.5 6 edges at (5, -19.0051, -49.4452) (5, -22.5051, -47.9452) (5, -22.5051, -50.9452) (5, -26.0051, -49.4452) (18, -19.0051, -47.9452) (18, -26.0051, -47.9452)
mirror "Mirror3" about plane through (5, 0, -52.5) normal (0, 1, 0) of "Fillet5", "Extrusion8", "Extrusion9"
sketch "Sketch36" plane through (5, 0, 0) normal (1, 0, 0) x (0, 0, -1)
  line L0 (50.9452, 19.0051) -> (48.4452, 19.0051) projected
  line L1 (50.9452, 19.0051) -> (5.4452, 19.0051)
  line L2 (5.4452, 19.0051) -> (5.4452, -3.2028)
  point P0 (0, 0)
  dimension "d67" = 45.5
  constraints: 4 end point, 1 horizontal, 1 perpendicular
  measures "d67" distance of L0.start L1.end
sketch "Sketch37" plane through (5, 0, 0) normal (1, 0, 0) x (0, 0, -1)
  point P0 (0, 0)
sketch "Sketch38" plane through (5, 0, 0) normal (1, 0, 0) x (0, 0, -1)
  point P0 (0, 0)
sketch "Sketch39" plane through (5, 0, 0) normal (1, 0, 0) x (0, 0, -1)
  point P0 (0, 0)
sketch "Sketch40" plane through (5, 0, -52.5) normal (0, 1, 0) x (0, 0, 1)
  line L0 (47.0548, 41.5507) -> (47.0548, -5)
  line L1 (106.5, -5) -> (-1.5, -5) projected
  line L2 (1.5548, 0.5) -> (1.5548, 26) projected
  point P0 (52.5, -5)
  dimension "d106" = 45.5
  constraints: 2 end point, 1 point on line, 1 vertical
  measures "d106" distance between parallel lines of L2 L0
sketch "Sketch41" plane through (5, 0, 0) normal (1, 0, 0) x (0, 0, -1)
  point P0 (0, 0)
sketch "Sketch42" plane through (5, 0, 0) normal (1, 0, 0) x (0, 0, -1)
  line L0 (51.6232, 18.4586) -> (-43.3768, 18.4586)
  point P0 (0, 0)
  dimension "d66" = 95
  constraints: 2 end point, 1 horizontal
  measures "d66" distance of L0.start L0.end
sketch "Sketch43" plane through (5, 0, 0) normal (1, 0, 0) x (0, 0, -1)
  point P0 (0, 0)
pattern_circular "Circular Pattern1" count 2 over 360 about axis through (46.5507, 0, -5.4452) along (-1, 0, 0) of "Fillet5", "Extrusion8", "Extrusion9", "Mirror3"
fillet "Fillet6" radius 0.5 3 edges at (5, -46.5, 0) (5, 0, 52.5) (18.55, -46.5, 52.5)
sketch "Sketch44" plane through (0, 0, 0) normal (-1, 0, 0) x (0, 0, 1)
  line L0 (-45.6543, 36.2401) -> (-46.9383, 39.7094)
  line L1 (-46.9383, 39.7094) -> (-44.0356, 42.0027)
  line L2 (-44.0356, 42.0027) -> (-40.9575, 39.9507)
  line L3 (-40.9575, 39.9507) -> (-41.958, 36.3892)
  line L4 (-41.958, 36.3892) -> (-45.6543, 36.2401)
  line L5 (-43.9087, 38.8584) -> (52.5, 38.8584)
  line L6 (52.5, 46.5) -> (52.5, -46) projected
  line L7 (-25.6543, 36.2401) -> (-26.9383, 39.7094)
  line L8 (-26.9383, 39.7094) -> (-24.0356, 42.0027)
  line L9 (-24.0356, 42.0027) -> (-20.9575, 39.9507)
  line L10 (-20.9575, 39.9507) -> (-21.958, 36.3892)
  line L11 (-21.958, 36.3892) -> (-25.6543, 36.2401)
  line L12 (-5.6543, 36.2401) -> (-6.9383, 39.7094)
  line L13 (-6.9383, 39.7094) -> (-4.0356, 42.0027)
  line L14 (-4.0356, 42.0027) -> (-0.9575, 39.9507)
  line L15 (-0.9575, 39.9507) -> (-1.958, 36.3892)
  line L16 (-1.958, 36.3892) -> (-5.6543, 36.2401)
  line L17 (14.3457, 36.2401) -> (13.0617, 39.7094)
  line L18 (13.0617, 39.7094) -> (15.9644, 42.0027)
  line L19 (15.9644, 42.0027) -> (19.0425, 39.9507)
  line L20 (19.0425, 39.9507) -> (18.042, 36.3892)
  line L21 (18.042, 36.3892) -> (14.3457, 36.2401)
  line L22 (34.3457, 36.2401) -> (33.0617, 39.7094)
  line L23 (33.0617, 39.7094) -> (35.9644, 42.0027)
  line L24 (35.9644, 42.0027) -> (39.0425, 39.9507)
  line L25 (39.0425, 39.9507) -> (38.042, 36.3892)
  line L26 (38.042, 36.3892) -> (34.3457, 36.2401)
  line L27 (-36.4027, 21.5316) -> (-37.6867, 25.0009)
  line L28 (-37.6867, 25.0009) -> (-34.7839, 27.2942)
  line L29 (-34.7839, 27.2942) -> (-31.7059, 25.2422)
  line L30 (-31.7059, 25.2422) -> (-32.7063, 21.6807)
  line L31 (-32.7063, 21.6807) -> (-36.4027, 21.5316)
  line L32 (-16.4027, 21.5316) -> (-17.6867, 25.0009)
  line L33 (-17.6867, 25.0009) -> (-14.7839, 27.2942)
  line L34 (-14.7839, 27.2942) -> (-11.7059, 25.2422)
  line L35 (-11.7059, 25.2422) -> (-12.7063, 21.6807)
  line L36 (-12.7063, 21.6807) -> (-16.4027, 21.5316)
  line L37 (3.5973, 21.5316) -> (2.3133, 25.0009)
  line L38 (2.3133, 25.0009) -> (5.2161, 27.2942)
  line L39 (5.2161, 27.2942) -> (8.2941, 25.2422)
  line L40 (8.2941, 25.2422) -> (7.2937, 21.6807)
  line L41 (7.2937, 21.6807) -> (3.5973, 21.5316)
  line L42 (23.5973, 21.5316) -> (22.3133, 25.0009)
  line L43 (22.3133, 25.0009) -> (25.2161, 27.2942)
  line L44 (25.2161, 27.2942) -> (28.2941, 25.2422)
  line L45 (28.2941, 25.2422) -> (27.2937, 21.6807)
  line L46 (27.2937, 21.6807) -> (23.5973, 21.5316)
  line L47 (43.5973, 21.5316) -> (42.3133, 25.0009)
  line L48 (42.3133, 25.0009) -> (45.2161, 27.2942)
  line L49 (45.2161, 27.2942) -> (48.2941, 25.2422)
  line L50 (48.2941, 25.2422) -> (47.2937, 21.6807)
  line L51 (47.2937, 21.6807) -> (43.5973, 21.5316)
  line L52 (-45.9428, 6.2374) -> (-47.2268, 9.7067)
  line L53 (-47.2268, 9.7067) -> (-44.3241, 12)
  line L54 (-44.3241, 12) -> (-41.2461, 9.948)
  line L55 (-41.2461, 9.948) -> (-42.2465, 6.3865)
  line L56 (-42.2465, 6.3865) -> (-45.9428, 6.2374)
  line L57 (-25.9428, 6.2374) -> (-27.2268, 9.7067)
  line L58 (-27.2268, 9.7067) -> (-24.3241, 12)
  line L59 (-24.3241, 12) -> (-21.2461, 9.948)
  line L60 (-21.2461, 9.948) -> (-22.2465, 6.3865)
  line L61 (-22.2465, 6.3865) -> (-25.9428, 6.2374)
  line L62 (-5.9428, 6.2374) -> (-7.2268, 9.7067)
  line L63 (-7.2268, 9.7067) -> (-4.3241, 12)
  line L64 (-4.3241, 12) -> (-1.2461, 9.948)
  line L65 (-1.2461, 9.948) -> (-2.2465, 6.3865)
  line L66 (-2.2465, 6.3865) -> (-5.9428, 6.2374)
  line L67 (14.0572, 6.2374) -> (12.7732, 9.7067)
  line L68 (12.7732, 9.7067) -> (15.6759, 12)
  line L69 (15.6759, 12) -> (18.7539, 9.948)
  line L70 (18.7539, 9.948) -> (17.7535, 6.3865)
  line L71 (17.7535, 6.3865) -> (14.0572, 6.2374)
  line L72 (34.0572, 6.2374) -> (32.7732, 9.7067)
  line L73 (32.7732, 9.7067) -> (35.6759, 12)
  line L74 (35.6759, 12) -> (38.7539, 9.948)
  line L75 (38.7539, 9.948) -> (37.7535, 6.3865)
  line L76 (37.7535, 6.3865) -> (34.0572, 6.2374)
  line L77 (-34.8195, -9.4352) -> (-36.1035, -5.9659)
  line L78 (-36.1035, -5.9659) -> (-33.2008, -3.6727)
  line L79 (-33.2008, -3.6727) -> (-30.1228, -5.7247)
  line L80 (-30.1228, -5.7247) -> (-31.1232, -9.2861)
  line L81 (-31.1232, -9.2861) -> (-34.8195, -9.4352)
  line L82 (-14.8195, -9.4352) -> (-16.1035, -5.9659)
  line L83 (-16.1035, -5.9659) -> (-13.2008, -3.6727)
  line L84 (-13.2008, -3.6727) -> (-10.1228, -5.7247)
  line L85 (-10.1228, -5.7247) -> (-11.1232, -9.2861)
  line L86 (-11.1232, -9.2861) -> (-14.8195, -9.4352)
  line L87 (5.1805, -9.4352) -> (3.8965, -5.9659)
  line L88 (3.8965, -5.9659) -> (6.7992, -3.6727)
  line L89 (6.7992, -3.6727) -> (9.8772, -5.7247)
  line L90 (9.8772, -5.7247) -> (8.8768, -9.2861)
  line L91 (8.8768, -9.2861) -> (5.1805, -9.4352)
  line L92 (25.1805, -9.4352) -> (23.8965, -5.9659)
  line L93 (23.8965, -5.9659) -> (26.7992, -3.6727)
  line L94 (26.7992, -3.6727) -> (29.8772, -5.7247)
  line L95 (29.8772, -5.7247) -> (28.8768, -9.2861)
  line L96 (28.8768, -9.2861) -> (25.1805, -9.4352)
  line L97 (45.1805, -9.4352) -> (43.8965, -5.9659)
  line L98 (43.8965, -5.9659) -> (46.7992, -3.6727)
  line L99 (46.7992, -3.6727) -> (49.8772, -5.7247)
  line L100 (49.8772, -5.7247) -> (48.8768, -9.2861)
  line L101 (48.8768, -9.2861) -> (45.1805, -9.4352)
  line L102 (-45.8331, -25.6371) -> (-47.1171, -22.1678)
  line L103 (-47.1171, -22.1678) -> (-44.2144, -19.8746)
  line L104 (-44.2144, -19.8746) -> (-41.1364, -21.9266)
  line L105 (-41.1364, -21.9266) -> (-42.1368, -25.488)
  line L106 (-42.1368, -25.488) -> (-45.8331, -25.6371)
  line L107 (-25.8331, -25.6371) -> (-27.1171, -22.1678)
  line L108 (-27.1171, -22.1678) -> (-24.2144, -19.8746)
  line L109 (-24.2144, -19.8746) -> (-21.1364, -21.9266)
  line L110 (-21.1364, -21.9266) -> (-22.1368, -25.488)
  line L111 (-22.1368, -25.488) -> (-25.8331, -25.6371)
  line L112 (-5.8331, -25.6371) -> (-7.1171, -22.1678)
  line L113 (-7.1171, -22.1678) -> (-4.2144, -19.8746)
  line L114 (-4.2144, -19.8746) -> (-1.1364, -21.9266)
  line L115 (-1.1364, -21.9266) -> (-2.1368, -25.488)
  line L116 (-2.1368, -25.488) -> (-5.8331, -25.6371)
  line L117 (14.1669, -25.6371) -> (12.8829, -22.1678)
  line L118 (12.8829, -22.1678) -> (15.7856, -19.8746)
  line L119 (15.7856, -19.8746) -> (18.8636, -21.9266)
  line L120 (18.8636, -21.9266) -> (17.8632, -25.488)
  line L121 (17.8632, -25.488) -> (14.1669, -25.6371)
  line L122 (34.1669, -25.6371) -> (32.8829, -22.1678)
  line L123 (32.8829, -22.1678) -> (35.7856, -19.8746)
  line L124 (35.7856, -19.8746) -> (38.8636, -21.9266)
  line L125 (38.8636, -21.9266) -> (37.8632, -25.488)
  line L126 (37.8632, -25.488) -> (34.1669, -25.6371)
  line L127 (10.1514, -39.0513) -> (9.151, -42.6128)
  line L128 (7.0734, -36.9993) -> (10.1514, -39.0513)
  line L129 (9.151, -42.6128) -> (5.4547, -42.7619)
  line L130 (4.1706, -39.2925) -> (7.0734, -36.9993)
  line L131 (-9.8486, -39.0513) -> (-10.849, -42.6128)
  line L132 (-12.9266, -36.9993) -> (-9.8486, -39.0513)
  line L133 (-10.849, -42.6128) -> (-14.5453, -42.7619)
  line L134 (-15.8294, -39.2925) -> (-12.9266, -36.9993)
  line L135 (-14.5453, -42.7619) -> (-15.8294, -39.2925)
  line L136 (5.4547, -42.7619) -> (4.1706, -39.2925)
  line L137 (-29.8486, -39.0513) -> (-30.849, -42.6128)
  line L138 (-32.9266, -36.9993) -> (-29.8486, -39.0513)
  line L139 (-30.849, -42.6128) -> (-34.5453, -42.7619)
  line L140 (-34.5453, -42.7619) -> (-35.8294, -39.2925)
  line L141 (-35.8294, -39.2925) -> (-32.9266, -36.9993)
  point P0 (0, 0)
  point P1 (-23.9087, 38.8584)
  point P2 (-3.9087, 38.8584)
  point P3 (16.0913, 38.8584)
  point P4 (36.0913, 38.8584)
  point P5 (-34.6571, 24.1499)
  point P6 (-14.6571, 24.1499)
  point P7 (5.3429, 24.1499)
  point P8 (25.3429, 24.1499)
  point P9 (45.3429, 24.1499)
  point P10 (-44.1972, 8.8557)
  point P11 (-24.1972, 8.8557)
  point P12 (-4.1972, 8.8557)
  point P13 (15.8028, 8.8557)
  point P14 (35.8028, 8.8557)
  point P15 (-33.0739, -6.8169)
  point P16 (-13.0739, -6.8169)
  point P17 (6.6375, -6.5284)
  point P18 (25.1805, -9.4352)
  point P19 (46.9261, -6.8169)
  point P20 (-44.0876, -23.0188)
  point P21 (-24.0876, -23.0188)
  point P22 (-4.0876, -23.0188)
  point P23 (15.9124, -23.0188)
  point P24 (35.9124, -23.0188)
  point P25 (7.2002, -40.1436)
  point P26 (-12.7998, -40.1436)
  point P27 (-32.7998, -40.1436)
  dimension "d74" = 20
  dimension "d83" = 20
  dimension "d88" = 20
  dimension "d93" = 20
  dimension "d98" = 20
  dimension "d103" = 20
  constraints: 282 end point, 2 horizontal, 1 coincident, 1 point on line, 110 other
  measures "d74" distance of L5.start point (-23.909, 38.858)
  measures "d83" distance of point (-34.657, 24.15) point (-14.657, 24.15)
  measures "d88" distance of point (-44.197, 8.856) point (-24.197, 8.856)
  measures "d93" distance of point (-33.074, -6.817) point (-13.074, -6.817)
  measures "d98" distance of point (-44.088, -23.019) point (-24.088, -23.019)
  measures "d103" distance of point (-32.8, -40.144) point (-12.8, -40.144)
extrude "Extrusion10" add sketch "Sketch44" along normal blind 1
sketch "Sketch45" plane through (5, 0, -52.5) normal (0, 1, 0) x (0, 0, 1)
  line L0 (47.0548, 57.8214) -> (47.0548, -23.4238) projected
  line L1 (47.0548, 41.5507) -> (47.0548, -5) projected
  line L2 (-1.5, 30) -> (106.5, 30) projected
  line L3 (90.0548, 0) -> (93.0548, 0) projected
  line L4 (89.0548, 0) -> (90.0548, 0) projected
  line L5 (90.0548, 0) -> (89.0548, 0) projected
  line L6 (93.0548, 0) -> (90.0548, 0) projected
  line L7 (4.0548, 0) -> (1.0548, 0) projected
  line L8 (5.0548, 0) -> (4.0548, 0) projected
  line L9 (4.0548, 0) -> (5.0548, 0) projected
  line L10 (1.0548, 0) -> (4.0548, 0) projected
  line L11 (0, 0) -> (104.5, 0) projected
  line L12 (104.5, 0) -> (0, 0) projected
  line L13 (4.0548, 0) -> (5.0548, 0) projected
  line L14 (1.0548, 0) -> (4.0548, 0) projected
  line L15 (4.0548, 0) -> (1.0548, 0) projected
  line L16 (5.0548, 0) -> (4.0548, 0) projected
  line L17 (90.0548, 0) -> (89.0548, 0) projected
  line L18 (93.0548, 0) -> (90.0548, 0) projected
  line L19 (90.0548, 0) -> (93.0548, 0) projected
  line L20 (89.0548, 0) -> (90.0548, 0) projected
  line L21 (48.0548, -11.8174) -> (48.0548, 46.215)
  point P0 (52.5, -5)
  point P1 (47.0548, 0)
  point P2 (47.0548, 0)
  point P3 (47.0548, 0)
  constraints: 2 end point, 1 vertical
sketch "Sketch46" plane through (1, -49, 55) normal (0, 0, 1) x (1, 0, 0)
  line L0 (33, 2.5) -> (34, 2.5) construction
  line L1 (33, 0) -> (31.1, 0) construction
  arc A0 (4, 3) -> (4.5, 2.5) centre (4.5, 3) ccw projected
  line L2 (31.1, 2.5) -> (4.5, 2.5) projected
  line L3 (31.1, 2.5) -> (31.1, 0) projected
  line L4 (31.1, 0) -> (33, 0) projected
  line L5 (33, 0) -> (33, 2.5) projected
  line L6 (34, 2.5) -> (33, 2.5) projected
  line L7 (34, 95.5519) -> (34, 2.5) projected
  line L8 (34, 95.5519) -> (33, 95.5519) projected
  line L9 (33, 95.5519) -> (33, 98) projected
  line L10 (33, 98) -> (31.1, 98) projected
  line L11 (31.1, 98) -> (31.1, 95.5) projected
  line L12 (31.1, 95.5) -> (4, 95.5) projected
  line L13 (4, 95.5) -> (4, 3) projected
  circle A1 centre (16.5, 49) radius 10.5 projected
  line L14 (34, 2.5) -> (34, 95.5519) projected
  point P0 (-1, 49)
  dimension "d107" = 2.5
  measures "d107" distance between parallel lines of L0 L1
sketch "Sketch47" plane through (0, 0, 0) normal (-1, 0, 0) x (0, 0, 1)
  point P0 (0, 0)
ref_plane "Work Plane4" through (32.5, 0, 0) normal (1, 0, 0) x (0, 0, -1)
body "Solid1"
